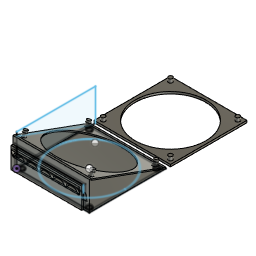
2022_12_25_MSI Pulse76 CPU Repalcement v5 (Autodesk Fusion 360 design; units mm, degrees)
Autodesk Fusion 360 part; units mm, degrees
sketch "Sketch1" plane through (0, 0, 0) normal (0, 0, 1) x (1, 0, 0)
  line L0 (0, 0) -> (76, 0)
  line L1 (76, 0) -> (76, 76)
  line L2 (76, 76) -> (0, 76)
  line L3 (0, 76) -> (0, 0)
  circle A0 centre (2.75, 73.25) radius 2.75
  circle A1 centre (73.25, 73.25) radius 2.75
  circle A2 centre (73.25, 2.75) radius 2.75
  circle A3 centre (2.75, 2.75) radius 2.75
  line L4 (-2, -2) -> (78, -2)
  line L5 (78, -2) -> (78, 78)
  line L6 (78, 78) -> (-2, 78)
  line L7 (-2, 78) -> (-2, -2)
  circle A4 centre (38, 38) radius 38
  circle A5 centre (38, 38) radius 37
  circle A6 centre (2.75, 73.25) radius 2.15
  circle A7 centre (73.25, 73.25) radius 2.15
  circle A8 centre (73.25, 2.75) radius 2.15
  circle A9 centre (2.75, 2.75) radius 2.15
  point P0 (17.79, 64.2008)
  dimension "d1" = 76
  dimension "d2" = 76
  dimension "d3" = 5.5
  dimension "d4" = 5.5
  dimension "d5" = 5.5
  dimension "d6" = 5.5
  dimension "d7" = 2
  dimension "d8" = -1
  dimension "d11" = -0.6
  dimension "d12" = -0.6
  dimension "d13" = -0.6
  dimension "d14" = -0.6
  constraint horizontal L0
  constraint vertical L1
  constraint horizontal L2
  constraint vertical L3
  constraint coincident L0.start L3.end
  constraint tangent L2 A0
  constraint tangent L3 A0
  constraint tangent L2 A1
  constraint tangent L1 A1
  constraint tangent L1 A2
  constraint tangent L0 A2
  constraint tangent L0 A3
  constraint tangent L3 A3
  constraint tangent L2 A4
  measures "d1" distance of L0.start L0.end
  measures "d2" distance of L0.start L2.end
  measures "d3" diameter of A0
  measures "d4" diameter of A1
  measures "d5" diameter of A2
  measures "d6" diameter of A3
extrude "Extrude1" add sketch "Sketch1" along normal blind 1.2 contours L0 L3 A3 | L0 L3 A3 A4 | A3 | L0 L1 A2 A4 | A4 | L2 L3 A0 A4 | L0 L1 A2 | A2 | L1 L2 A1 A4 | L2 L3 A0 | A0 | L1 L2 A1 | A1 | L4 L5 L6 L7 | A6 | A7 | A8 | A9 makes body 1
extrude "Extrude2" add sketch "Sketch1" along normal blind 5 contours A6 | A7 | A8 | A9 bodies 1
move_body "Move1" bodies 1 to x (1, 0, 0) y (0, 0.996195, -0.087156) z (0, 0.087156, 0.996195) at (0, 0.2968, 6.7981)
sketch "Sketch2" plane through (0, 0, 0) normal (0, 1, 0) x (1, 0, 0)
  line L0 (0, 0) -> (70, 0)
  line L1 (70, 0) -> (70, -20)
  line L2 (70, -20) -> (0, -20)
  line L3 (0, -20) -> (0, 0)
  line L4 (0, -20) -> (70, -20)
  line L5 (70, -20) -> (70, -13)
  line L6 (70, -13) -> (0, -13)
  line L7 (0, -13) -> (0, -20)
  line L8 (-2, -22) -> (-2, 0)
  line L9 (72, 0) -> (72, -22)
  line L10 (72, -22) -> (-2, -22)
  line L11 (-2, 0) -> (0, 0)
  line L12 (70, 0) -> (72, 0)
  line L13 (0, -13) -> (70, -13)
  line L14 (70, -13) -> (70, -20)
  line L15 (70, -20) -> (0, -20)
  line L16 (0, -20) -> (0, -13)
  line L17 (0.5, -19.5) -> (0.5, -13.5)
  line L18 (69.5, -13.5) -> (0.5, -13.5)
  line L19 (69.5, -19.5) -> (69.5, -13.5)
  line L20 (69.5, -19.5) -> (0.5, -19.5)
  dimension "d18" = 70
  dimension "d19" = 20
  dimension "d20" = 7
  dimension "d25" = 0.5
  constraint horizontal L0
  constraint vertical L1
  constraint horizontal L2
  constraint vertical L3
  constraint coincident L0.start L3.end
  constraint horizontal L4
  constraint vertical L5
  constraint horizontal L6
  constraint vertical L7
  constraint perpendicular L3 L11
  constraint perpendicular L9 L12
  constraint horizontal L13
  constraint vertical L14
  constraint horizontal L15
  constraint vertical L16
  measures "d18" distance of L0.start L0.end
  measures "d19" distance of L0.start L2.end
  measures "d20" distance of L2.end L6.end
extrude "Extrude3" add sketch "Sketch2" against normal blind 4 separate body contours L0 L1 L3 L6 L13 | L1 L2 L3 L4 L5 L7 L8 L9 L10 L11 L12 L14 L15 L16 makes body 2
move_body "Move2" bodies 1 to x (1, 0, 0) y (0, 0.965926, -0.258819) z (0, 0.258819, 0.965926) at (0, 2.6578, 20.1879)
extrude "Extrude4" add sketch "Sketch2" against normal blind 6 contours L1 L2 L3 L4 L5 L6 L7 L13 L14 L15 L16 bodies 2
sketch "Sketch3" plane through (0, 0, 0) normal (1, 0, 0) x (0, 1, 0)
  line L0 (0, 0) -> (82.4686, 0)
  line L1 (82.4686, 0) -> (82.4686, 33.3706)
  line L2 (82.4686, 33.3706) -> (0, 33.3706)
  line L3 (0, 33.3706) -> (0, 0)
  line L4 (78, 0) -> (0, 29)
  constraint horizontal L0
  constraint vertical L1
  constraint horizontal L2
  constraint vertical L3
  constraint coincident L0.start L3.end
  constraint coincident L0 L4.start
  constraint coincident L3 L4.end
extrude "Extrude5" add sketch "Sketch1" along normal blind 30 separate body contours L4 L5 L6 L7 makes body 3
extrude "Extrude6" cut sketch "Sketch3" along normal blind 108 and the other way blind 15 contours L0 L1 L2 L3 L4 bodies 3
move_body "Move3" bodies 1 to x (1, 0, 0) y (0, 1, 0) z (0, 0, 1) at (0, -3, 1)
extrude "Extrude7" add 1 faces at (51.3333, 75.2736, 1.7518) along direction (0, 0.939693, -0.34202) blind 3 separate body on bodies 1 makes body 4
extrude "Extrude8" cut sketch "Sketch2" against normal blind 23 contours L17 L18 L19 L20 bodies 3
combine "Combine1" operation cut target body 3 tool bodies 1 keep tools
move_body "Move4" bodies 1 to x (1, 0, 0) y (0, 1, 0) z (0, 0, 1) at (0, 0, 9)
extrude "Extrude9" add 1 faces at (50.6667, 76, 0.2479) along direction (0, -1, 0) blind 78 on bodies 3 bodies 3 2 4
draft "Draft1" angle -5 neutral plane through (0, -4, 0) pull (0, -1, 0) 1 faces at (46.5, -2, 13.5) on bodies 3
draft "Draft2" angle 10 neutral plane through (0, -4, 0) pull (0, -1, 0) 1 faces at (46.6667, -4.6667, 13) on bodies 3
copy_body "CopyPasteBodies1" bodies 1 makes body 5
move_body "Move5" bodies 5 to x (1, 0, 0) y (0, 1, 0) z (0, 0, 1) at (0, 90, 0)
move_body "Move6" bodies 5 to x (1, 0, 0) y (0, 0.939693, 0.34202) z (0, -0.34202, 0.939693) at (0, 13.3709, -55.8302)
move_body "Move7" bodies 5 to x (1, 0, 0) y (0, 1, 0) z (0, 0, 1) at (0, -87, -10)
move_body "Move8" bodies 5 to x (1, 0, 0) y (0, 1, 0) z (0, 0, 1) at (0, 85, 0)
sketch "Sketch4" plane through (0, 0, 0) normal (0, 1, 0) x (1, 0, 0)
extrude "Extrude10" add 1 faces at (7.936, 91.6353, 0) along direction (0, 0, -1) blind 1 on bodies 5 bodies 5
move_body "Move9" bodies 1 to x (1, 0, 0) y (0, 1, 0) z (0, 0, 1) at (0, 0, -9)
extrude "Extrude11" add 4 faces at (2.4882, 72.7861, 7.1267) (72.6961, 71.72, 7.5147) (72.6961, 6.5248, 31.2438) (3.5254, 5.2612, 31.7037) along direction (0, 0.34202, 0.939693) blind 2 separate body on bodies 1 makes body 6 at (72.8767, 8.4439, 31.9642) makes body 7 at (4.8973, 72.5753, 7.9129) makes body 8 at (72.9827, 74.4792, 7.2199) makes body 9 at (4.8893, 6.0251, 32.1352)
extrude "Extrude12" add 4 faces at (3.5254, 5.2612, 31.7037) (72.6961, 6.5248, 31.2438) (72.6961, 71.72, 7.5147) (2.4882, 72.7861, 7.1267) along direction (0, -0.34202, -0.939693) blind 10 on bodies 6 7 8 9 bodies 9 3 6 7 8
extrude "Extrude13" add 2 faces at (72.6961, 7.2088, 33.1232) (3.5254, 5.9452, 33.5831) along direction (0, -0.34202, -0.939693) blind 26 separate body on bodies 6 9 makes body 10 at (72.9827, 5.7228, 24.4412) makes body 11 at (4.8973, 0.6532, 17.0635)
extrude "Extrude14" cut 1 faces at (49.3333, -2, 27.3333) along direction (0, -1, 0) blind 4 on bodies 3 bodies 10
extrude "Extrude15" cut 1 faces at (46.6667, -4, 4.3333) along direction (0, -1, 0) blind 1 on bodies 3 bodies 11
extrude "Extrude16" cut sketch "Sketch1" against normal blind 6 contours A4 | L2 L3 A0 A4 | L1 L2 A1 A4 | A0 | A1 | A5 | A6 | A7 bodies 3
sketch "Sketch5" plane through (0, 0, 0) normal (0, 1, 0) x (1, 0, 0)
  line L0 (0.5, -13.5) -> (69.5, -13.5)
  line L1 (69.5, -13.5) -> (69.5, -19.5)
  line L2 (69.5, -19.5) -> (0.5, -19.5)
  line L3 (0.5, -19.5) -> (0.5, -13.5)
  line L4 (1.1304, -13.5) -> (13.1304, -13.5)
  arc A0 (1.1304, -13.5) -> (13.1304, -13.5) centre (7.1304, -13.5) ccw
  line L5 (7.1304, -13.5) -> (7.1304, -14)
  line L6 (7.1304, -14) -> (7.1304, -19.5)
  arc A1 (14.8804, -13.5) -> (26.8804, -13.5) centre (20.8804, -13.5) ccw
  arc A2 (28.6304, -13.5) -> (40.6304, -13.5) centre (34.6304, -13.5) ccw
  arc A3 (42.3804, -13.5) -> (54.3804, -13.5) centre (48.3804, -13.5) ccw
  arc A4 (56.1304, -13.5) -> (68.1304, -13.5) centre (62.1304, -13.5) ccw
  point P0 (0.5, -13.5)
  point P1 (69.5, -19.5)
  dimension "d73" = 55
  dimension "d74" = 0
  constraint horizontal L0
  constraint vertical L1
  constraint horizontal L2
  constraint vertical L3
  constraint coincident P1 L1.end
  constraint coincident P0 L0.start
  constraint coincident L0 A0.centre
  constraint tangent L2 A0
  constraint coincident L0 L4.start
  constraint coincident L0 L4.end
  constraint coincident A0.centre L5.start
  constraint perpendicular L4 L5
  constraint midpoint A0 L6.end
  constraint perpendicular L2 L6
extrude "Extrude17" add sketch "Sketch5" against normal blind 6 contours L0 L2 L3 A0 | L0 L2 A0 A1 | L0 L2 A1 A2 | L0 L2 A2 A3 | L0 L2 A3 A4 | L0 L1 L2 A4 bodies 3 11
extrude "Extrude18" cut 1 faces at (33.73, -1.3333, 13.2667) along direction (0, -0.087156, -0.996195) blind 1 on bodies 3 bodies 3
extrude "Extrude19" add 1 faces at (47.9667, -1.6037, 12.2865) along direction (0, 0.087156, 0.996195) blind 1.3 on bodies 3 bodies 3
draft "Draft3" angle -15 neutral plane through (70, 0, 20) pull (0, 0, 1) 1 faces at (69.2735, -6, 16.252) on bodies 3
